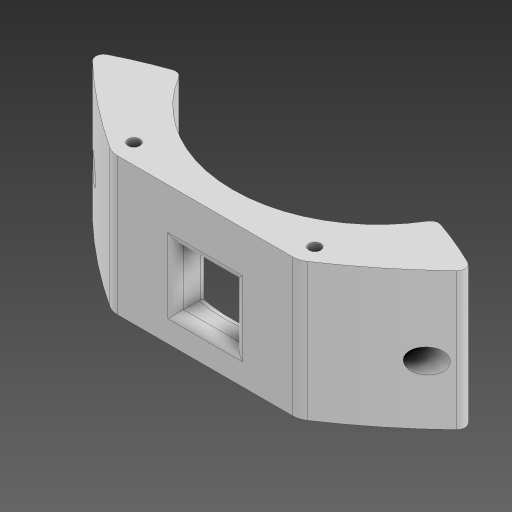
# Autodesk Inventor part: ball_solenoid
Saved by Autodesk Inventor 2023 (Build 270158000, 158)
## iProperties
Created: 2025-06-23
Part Number: ball_solenoid
Material: Типовые
Document SubType Name: Modeling
Designer: daa
Density: 1 g/cm^3
Appearance: По умолчанию
Author: daa
Autodesk Inventor part; units mm, degrees
ref_plane "YZ Plane" through (0, 0, 0) normal (1, 0, 0) x (0, 1, 0)
ref_plane "XZ Plane" through (0, 0, 0) normal (0, 1, 0) x (-1, 0, 0)
ref_plane "XY Plane" through (0, 0, 0) normal (0, 0, 1) x (1, 0, 0)
sketch "Эскиз1" plane through (0, 0, 0) normal (0, 1, 0) x (-1, 0, 0)
  line L0 (-22.4119, 54.6751) -> (22.1979, 54.6751)
  arc A0 (32.489, 28.2049) -> (-32.489, 28.2049) centre (0, 10.5) ccw
  arc A1 (36.6633, -21.4663) -> (-36.0003, -21.4663) centre (0.3315, -28.4663) ccw
  line L1 (36.6633, -21.4663) -> (-36.0003, -21.4663)
  circle A2 centre (23, 49.6751) radius 1.5
  arc A3 (32.489, 28.2049) -> (48.2755, 35.0087) centre (-0.6395, 126.7874) ccw
  circle A4 centre (-23, 49.6751) radius 1.5
  arc A5 (-48.2758, 34.8835) -> (-32.489, 28.2049) centre (0, 127) ccw
  arc A6 (-25.1833, 53.8367) -> (-48.2758, 34.8835) centre (57.9612, -71.0112) ccw
  arc A7 (48.2755, 35.0087) -> (24.9347, 53.8596) centre (-57.1689, -71.6753) ccw
  arc A8 (24.9347, 53.8596) -> (22.1979, 54.6751) centre (22.1979, 49.6751) ccw
  arc A9 (-22.4119, 54.6751) -> (-25.1833, 53.8367) centre (-22.4119, 49.6751) ccw
  point P0 (0, 0)
  point P1 (0, 0)
  point P2 (-23.9104, 54.6751)
  point P3 (0, 47.5)
  point P4 (-0.107, 54.6751)
  point P5 (0, 0)
  point P6 (23.6741, 54.6751)
  dimension "d0" = 72.6636
  dimension "d1" = 37
  dimension "d2" = 15.7868
  dimension "d3" = 7.1751
  dimension "d4" = 5
  dimension "d5" = 5
  dimension "d6" = 150
  dimension "d7" = 150
  dimension "d8" = 5
  dimension "d95" = 23
  dimension "d96" = 23
  constraints: 19 point on circle, 10 centre point, 4 end point, 4 tangent, 2 horizontal, 2 point on line, 1 equal radius, 1 midpoint
  measures "d0" distance of L1.start L1.end
  measures "d1" radius of A1
  measures "d2" horizontal distance of A6.end A5.end
  measures "d3" vertical distance of point (-0.107, 54.675) point (0, 47.5)
  measures "d4" vertical distance of point (23.674, 54.675) A2.centre
  measures "d5" vertical distance of point (-23.91, 54.675) A4.centre
  measures "d6" radius of A6
  measures "d7" radius of A7
  measures "d8" radius of A8
  measures "d95" horizontal distance of point (0, 47.5) A2.centre
  measures "d96" horizontal distance of A4.centre point (0, 47.5)
extrude "Выдавливание1" add sketch "Эскиз1" along normal blind 35 contours L0 A8 A7 A3 A0 A5 A6 A9
sketch "Эскиз7" plane through (-22.1979, 0, 54.6751) normal (0, 0, 1) x (1, 0, 0)
  line L0 (14.805, 22.5) -> (29.805, 22.5)
  line L1 (29.805, 22.5) -> (29.805, 7.5)
  line L2 (29.805, 7.5) -> (14.805, 7.5)
  line L3 (14.805, 7.5) -> (14.805, 22.5)
  line L4 (0, 35) -> (44.6098, 35) projected
  line L5 (0, 0) -> (0, 35) projected
  point P0 (22.1979, 0)
  dimension "d40" = 15
  dimension "d41" = 15
  dimension "d42" = 12.5
  dimension "d43" = 14.805
  constraints: 8 end point, 2 parallel, 1 horizontal, 1 perpendicular
  measures "d40" distance of L1.end L2.end
  measures "d41" distance of L0.end L1.end
  measures "d42" distance between parallel lines of L4 L0
  measures "d43" distance between parallel lines of L5 L3
extrude "Выдавливание5" cut sketch "Эскиз7" against normal blind 48
fillet "Сопряжение1" radius 2 8 edges at (0.1071, 7.5, 54.6751) (-7.3929, 15, 54.6751) (0.1071, 22.5, 54.6751) (7.6071, 15, 54.6751) (7.6071, 15, 46.7096) (0.1093, 22.5, 47.4998) (-7.3929, 15, 46.7539) (0.1093, 7.5, 47.4998)
fillet "Сопряжение2" radius 2 4 edges at (48.2758, 17.5, 34.8835) (32.489, 17.5, 28.2049) (-32.489, 17.5, 28.2049) (-48.2755, 17.5, 35.0087)
ref_plane "РабПлоскость4" through (34.061, 0, 28.7358) normal (0.3275101, 0, -0.9448477) x (0, 1, 0)
sketch "Эскиз9" plane through (34.061, 0, 28.7358) normal (0.3275101, 0, -0.9448477) x (0, 1, 0)
  circle A0 centre (25, 6.331) radius 2
  circle A1 centre (5, 6.331) radius 2
  line L0 (35, 0) -> (35, 12.662) projected
  line L1 (0, 12.662) -> (35, 12.662) projected
  point P0 (0, -41.5938)
  dimension "d49" = 4
  dimension "d50" = 4
  dimension "d51" = 20
  dimension "d52" = 10
  dimension "d53" = 6.331
  dimension "d54" = 6.331
  constraints: 2 centre point
  measures "d49" diameter of A0
  measures "d50" diameter of A1
  measures "d51" distance of A1.centre A0.centre
  measures "d52" distance from line of A0.centre L0
  measures "d53" distance from line of A0.centre L1
  measures "d54" distance from line of L1 A1.centre
extrude "Выдавливание6" cut sketch "Эскиз9" against normal blind 10
ref_plane "РабПлоскость9" through (-46.1693, 0, 32.8004) normal (0.3907574, 0, 0.9204937) x (0, -1, 0)
ref_plane "РабПлоскость8" through (-45.7785, 0, 33.7209) normal (0.3907574, 0, 0.9204937) x (0, -1, 0)
sketch "Эскиз12" plane through (-46.1693, 0, 32.8004) normal (0.3907574, 0, 0.9204937) x (0, -1, 0)
  circle A0 centre (-25, 6.3912) radius 2
  circle A1 centre (-5, 6.3912) radius 2
  line L0 (0, 12.7222) -> (-35, 12.7222) projected
  line L1 (-35, 12.7222) -> (-35, 0) projected
  point P0 (0, 55.3155)
  dimension "d66" = 4
  dimension "d67" = 4
  dimension "d68" = 20
  dimension "d69" = 6.331
  dimension "d70" = 6.331
  dimension "d71" = 10
  constraints: 2 centre point
  measures "d66" diameter of A0
  measures "d67" diameter of A1
  measures "d68" distance of A1.centre A0.centre
  measures "d69" distance from line of A0.centre L0
  measures "d70" distance from line of A1.centre L0
  measures "d71" distance from line of L1 A0.centre
extrude "Выдавливание8" cut sketch "Эскиз12" along normal blind 10
ref_plane "РабПлоскость12" through (46.281, 0, 36.8478) normal (-0.9961947, 0, -0.0871557) x (0, -1, 0)
sketch "Эскиз14" plane through (46.281, 0, 36.8478) normal (-0.9961947, 0, -0.0871557) x (0, -1, 0)
  circle A0 centre (-15, 4) radius 3.1
  line L0 (0, 18.763) -> (0, 0) projected
  line L1 (-35, 0) -> (0, 0) projected
  point P0 (0, -32.6739)
  dimension "d78" = 6.2
  dimension "d79" = 15
  dimension "d80" = 4
  constraints: 1 centre point
  measures "d78" diameter of A0
  measures "d79" distance from line of A0.centre L0
  measures "d80" distance from line of L1 A0.centre
extrude "Выдавливание9" cut sketch "Эскиз14" along normal blind 43.25
ref_plane "РабПлоскость13" through (-46.265, 0, 36.9591) normal (-0.9947346, 0, 0.1024849) x (0, 1, 0)
sketch "Эскиз16" plane through (-46.265, 0, 36.9591) normal (-0.9947346, 0, 0.1024849) x (0, 1, 0)
  circle A0 centre (15, -4) radius 3
  line L0 (0, -18.9975) -> (0, 0) projected
  line L1 (0, 0) -> (35, 0) projected
  point P0 (0, 32.0231)
  dimension "d85" = 6
  dimension "d86" = 15
  dimension "d87" = 4
  constraints: 1 centre point
  measures "d85" diameter of A0
  measures "d86" distance from line of L0 A0.centre
  measures "d87" distance from line of A0.centre L1
extrude "Выдавливание10" cut sketch "Эскиз16" against normal blind 19.25
sketch "Эскиз17" plane through (-46.265, 0, 36.9591) normal (-0.9947346, 0, 0.1024849) x (0, 1, 0)
  circle A0 centre (15, -4) radius 1.25
  line L0 (0, -18.9975) -> (0, 0) projected
  line L1 (0, 0) -> (35, 0) projected
  point P0 (0, 32.0231)
  dimension "d90" = 2.5
  dimension "d91" = 15
  dimension "d92" = 4
  constraints: 1 centre point
  measures "d90" diameter of A0
  measures "d91" distance from line of L0 A0.centre
  measures "d92" distance from line of A0.centre L1
extrude "Выдавливание11" cut sketch "Эскиз17" against normal blind 26.5
